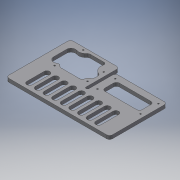
# Autodesk Inventor part: Plataforma
Saved by Autodesk Inventor 2017 (Build 210142000, 142)
## iProperties
Created: 2019-04-18
Part Number: Plataforma
Material: Generic
Document SubType Name: Modeling
Designer: Marcus
Density: 1 g/cm^3
Appearance: Default
CONJUNTO: TEXTO CONJUNTO
EQUIPAMENTO: TEXTO EQUIPAMENTO
SUBCONJUNTO: TEXTO SUBCONJUNTO
Author: Marcus
Autodesk Inventor part; units mm, degrees
sketch "Sketch1" plane through (0, 0, 0) normal (0, 0, 1) x (1, 0, 0)
  line L0 (90, -26) -> (-90, -26)
  line L1 (-90, -26) -> (-90, 26)
  line L2 (-90, 26) -> (90, 26)
  line L3 (90, 26) -> (90, -26)
  line L4 (90, -26) -> (-90, 26) construction
  line L5 (-90, -26) -> (90, 26) construction
  line L6 (-5, -26) -> (-90, -26)
  line L7 (-90, -26) -> (-90, -86)
  line L8 (-90, -86) -> (-5, -86)
  line L9 (-5, -86) -> (-5, -26)
  point P0 (0, 0)
  dimension "d2" = 180
  dimension "d3" = 52
  dimension "d6" = 85
  dimension "d7" = 60
  dimension "d8" = 0
  constraints: 20 end point, 4 parallel, 2 horizontal, 2 midpoint, 2 perpendicular, 1 point on line
  measures "d2" distance of L0.start L0.end
  measures "d3" distance of L2.end L0.start
  measures "d6" distance of L8.end L7.end
  measures "d7" distance of L7.end L6.end
  measures "d8" distance between parallel lines of L1 L7
extrude "Extrusion1" add sketch "Sketch1" along normal blind 6
ref_plane "Work Plane1" through (0, -29.4202, -0.6031) normal (0, 0.3420201, -0.9396926) x (-1, 0, 0)
sketch "Sketch4" plane through (0, 0, 0) normal (0, 0, -1) x (-1, 0, 0)
  circle A0 centre (12.2, -66.1) radius 1.6 projected
  circle A1 centre (63.1, -81.4) radius 1.6 projected
  circle A2 centre (64.6, -33.1) radius 1.6 projected
  circle A3 centre (12.2, -38) radius 1.6 projected
  point P0 (0, 27.8522)
  constraints: 4 coincident
hole "Hole2" at (-63.1, -81.4, 0) at (-12.2, -66.1, 0) at (-12.2, -38, 0) at (-64.6, -33.1, 0) direction (0, 0, 1) diameter 2.5 end through all
sketch "Sketch5" plane through (0, 0, 6) normal (0, 0, 1) x (1, 0, 0)
  line L0 (-5, -26) -> (90, -26) projected
  line L1 (0, -26) -> (90, -26)
  line L2 (90, -26) -> (90, -74)
  line L3 (90, -74) -> (0, -74)
  line L4 (0, -74) -> (0, -26)
  point P0 (0, 0)
  dimension "d25" = 90
  dimension "d26" = 0
  dimension "d27" = 48
  constraints: 8 end point, 2 parallel, 1 horizontal, 1 perpendicular, 1 point on line
  measures "d25" distance of L2.end L3.end
  measures "d26" distance from line of L0.end L2
  measures "d27" distance of L1.end L2.end
extrude "Extrusion2" add sketch "Sketch5" against normal blind 6
ref_plane "Work Plane4" through (95, -30.2262, -0.9369) normal (0, 0.4226183, -0.9063078) x (-1, 0, 0)
sketch "Sketch7" plane through (0, 0, 0) normal (0, 0, -1) x (-1, 0, 0)
  line L0 (-90, -74) -> (0, -74) projected
  line L1 (0, -74) -> (0, -26) projected
  point P0 (95, 27.7902)
  point P1 (-8, -66)
  point P2 (-83, -66)
  point P3 (-83, -35)
  point P4 (-8, -35)
  dimension "d32" = 75
  dimension "d33" = 31
  dimension "d68" = 8
  dimension "d69" = 8
  constraints: 2 horizontal alignment, 2 vertical alignment
  measures "d32" distance of point (-83, -66) point (-8, -66)
  measures "d33" distance of point (-8, -35) point (-8, -66)
  measures "d68" distance from line of L0 point (-8, -66)
  measures "d69" distance from line of L1 point (-8, -66)
hole "Hole3" at (8, -66, 0) at (83, -66, 0) at (83, -35, 0) at (8, -35, 0) direction (0, 0, 1) diameter 2.5 end through all
sketch "Sketch8" plane through (0, 0, 0) normal (0, 0, -1) x (-1, 0, 0)
  line L0 (5, -20) -> (-5, -20)
  line L1 (-5, -20) -> (-5, 20)
  line L2 (-5, 20) -> (5, 20)
  line L3 (5, 20) -> (5, -20)
  line L4 (5, -20) -> (-5, 20) construction
  line L5 (-5, -20) -> (5, 20) construction
  point P0 (0, 0)
  dimension "d43" = 10
  dimension "d44" = 40
  constraints: 12 end point, 2 midpoint, 2 parallel, 1 horizontal, 1 perpendicular
  measures "d43" distance of L1.end L2.end
  measures "d44" distance of L0.end L1.end
extrude "Extrusion3" cut sketch "Sketch8" against normal through all
fillet "Fillet1" radius 5 4 edges at (-5, -20, 3) (5, -20, 3) (-5, 20, 3) (5, 20, 3)
pattern_linear "Rectangular Pattern1" count 5 spacing 15 along (-1, 0, 0) of "Extrusion3", "Fillet1"
mirror "Mirror1" about plane through (0, 0, 0) normal (1, 0, 0) of "Extrusion3", "Rectangular Pattern1", "Fillet1"
ref_plane "Work Plane2" through (0, -29.4202, 0) normal (0, 0, -1) x (-1, 0, 0)
sketch "Sketch9" plane through (0, -29.4202, 0) normal (0, 0, -1) x (-1, 0, 0)
  arc A0 (23.024, -47.3212) -> (14.2141, -29.941) centre (8.7697, -43.6237) ccw
  arc A1 (23.024, -47.3212) -> (26.9699, -51.6786) centre (26.4278, -48.2041) ccw
  line L0 (26.9699, -51.6786) -> (50.5257, -51.6786)
  arc A2 (68.0822, -45.8989) -> (56.4491, -48.2055) centre (64.2405, -57.0121) ccw
  arc A3 (68.0822, -45.8989) -> (78.6732, -39.9653) centre (70.7371, -38.2188) ccw
  line L1 (78.6732, -39.9653) -> (78.6732, -15.7542)
  arc A4 (78.6732, -15.7542) -> (66.1708, -9.0999) centre (70.6511, -15.7542) ccw
  arc A5 (59.4126, -7.792) -> (66.1708, -9.0999) centre (63.4478, -5.0555) ccw
  line L2 (55.2743, -5.5982) -> (23.1432, -5.5982)
  arc A6 (14.3811, -15.6329) -> (18.1453, -10.453) centre (12.4723, -10.2882) ccw
  line L3 (11.0627, -20.3417) -> (11.0627, -25.2953)
  arc A7 (53.6862, -50.553) -> (56.4491, -48.2055) centre (-3.5207, 19.5774) ccw
  arc A8 (59.4126, -7.792) -> (55.2743, -5.5982) centre (55.2743, -10.5982) ccw
  arc A9 (23.1432, -5.5982) -> (18.1453, -10.453) centre (23.1432, -10.5982) ccw
  arc A10 (14.3811, -15.6329) -> (11.0627, -20.3417) centre (16.0627, -20.3417) ccw
  arc A11 (11.0627, -25.2953) -> (14.2141, -29.941) centre (16.0627, -25.2953) ccw
  arc A12 (50.5257, -51.6786) -> (53.6862, -50.553) centre (50.5257, -46.6786) ccw
  point P0 (0, 27.8522)
  point P1 (11.0627, -29.0773)
  point P2 (58.6025, -5.5982)
  point P3 (15.6681, -5.5982)
  point P4 (52.2779, -51.6786)
  point P5 (52.2779, -51.6786)
  dimension "d51" = 5
  dimension "d85" = 5
  constraints: 31 point on circle, 15 tangent, 13 centre point, 8 end point, 5 point on line, 3 equal radius, 2 horizontal, 1 vertical
  measures "d51" radius of A8
  measures "d85" radius of A12
extrude "Extrusion4" cut sketch "Sketch9" against normal blind 6
ref_plane "Work Plane3" through (90, -74, 0) normal (0, 0, 1) x (-1, 0, 0)
sketch "Sketch10" plane through (90, -74, 0) normal (0, 0, 1) x (-1, 0, 0)
  line L0 (72, -36) -> (17, -36)
  line L1 (12, -31) -> (12, -16)
  line L2 (17, -11) -> (72, -11)
  line L3 (77, -16) -> (77, -31)
  arc A0 (72, -36) -> (77, -31) centre (72, -31) ccw
  arc A1 (77, -16) -> (72, -11) centre (72, -16) ccw
  arc A2 (17, -11) -> (12, -16) centre (17, -16) ccw
  arc A3 (12, -31) -> (17, -36) centre (17, -31) ccw
  circle A4 centre (82, -8) radius 1.25 projected
  circle A5 centre (7, -8) radius 1.25 projected
  circle A6 centre (7, -39) radius 1.25 projected
  point P0 (95, 27.7902)
  dimension "d54" = 5
  dimension "d71" = 25
  dimension "d72" = 65
  dimension "d73" = 75
  dimension "d74" = 5
  dimension "d76" = 31
  dimension "d77" = 3
  constraints: 8 end point, 8 point on circle, 8 tangent, 4 centre point, 3 equal radius, 2 parallel, 1 horizontal, 1 perpendicular
  measures "d54" radius of A0
  measures "d71" distance between parallel lines of L0 L2
  measures "d72" distance between parallel lines of L1 L3
  measures "d73" distance of A5.centre A4.centre
  measures "d74" distance from line of A4.centre L3
  measures "d76" distance of A6.centre A5.centre
  measures "d77" distance from line of A5.centre L2
extrude "Extrusion5" cut sketch "Sketch10" along normal blind 6 contours L0 A3 L1 A2 L2 A1 L3 A0
fillet "Fillet2" radius 5 6 edges at (90, 26, 3) (-90, 26, 3) (90, -74, 3) (0, -74, 3) (-5, -86, 3) (-90, -86, 3)
sketch "Sketch13" plane through (0, 0, 6) normal (0, 0, 1) x (1, 0, 0)
  circle A0 centre (83, -66) radius 1.25 projected
  circle A1 centre (83, -35) radius 1.25 projected
  circle A2 centre (8, -35) radius 1.25 projected
  circle A3 centre (8, -66) radius 1.25 projected
  circle A4 centre (-12.2, -66.1) radius 1.25 projected
  circle A5 centre (-12.2, -38) radius 1.25 projected
  circle A6 centre (-64.6, -33.1) radius 1.25 projected
  circle A7 centre (-63.1, -81.4) radius 1.25 projected
  point P0 (0, 0)
  constraints: 8 coincident
hole "Hole4" at (83, -66, 6) at (8, -66, 6) at (8, -35, 6) at (83, -35, 6) at (-12.2, -38, 6) at (-12.2, -66.1, 6) at (-63.1, -81.4, 6) at (-64.6, -33.1, 6) direction (0, 0, -1) diameter 6 depth 3
fillet "Fillet3" radius 2 2 edges at (-5, -26, 3) (0, -26, 3)
equation "\"d74\" = -0.5 * d72 + 0.5 * d73"
equation "\"d77\" = -0.5 * d71 + 0.5 * d76"
body "Solid1"
